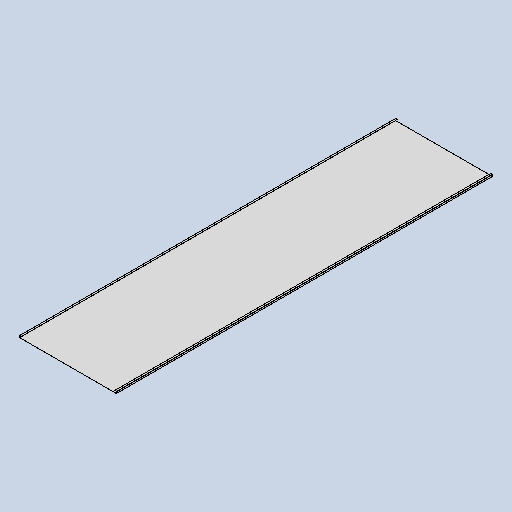
# Autodesk Inventor part: MSC 812 sheet gills
Saved by Autodesk Inventor 2025 (Build 290162010, 162A)
## iProperties
Created: 2024-06-15
Part Number: MSC 812 sheet gills
Material: Stainless Steel
Document SubType Name: Sheet Metal
Designer: pokla
Stock Number: МОО 0101 лист жабра
Mass: 8000 g
Surface Area: 40030 cm^2
Volume: 1000 cm^3
Density: 8 g/cm^3
Sheet Metal Rule: Default_mm
Appearance: Default
Author: pokla
Autodesk Inventor part; units mm, degrees
ref_plane "YZ Plane" through (0, 0, 0) normal (1, 0, 0) x (0, 1, 0)
ref_plane "XZ Plane" through (0, 0, 0) normal (0, 1, 0) x (-1, 0, 0)
ref_plane "XY Plane" through (0, 0, 0) normal (0, 0, 1) x (1, 0, 0)
sketch "Sketch6" plane through (0, 0, 0) normal (0, 1, 0) x (-1, 0, 0)
  line L0 (255.9, -990) -> (-255.9, -990)
  line L1 (-255.9, -990) -> (-255.9, 990)
  line L2 (-255.9, 990) -> (255.9, 990)
  line L3 (255.9, 990) -> (255.9, -990)
  line L4 (255.9, -990) -> (-255.9, 990) construction
  line L5 (-255.9, -990) -> (255.9, 990) construction
  point P0 (0, 0)
  dimension "d52" = 511.8
  dimension "d53" = 1980
  measures "d52" distance of L1.end L2.end
  measures "d53" distance of L0.end L1.end
extrude "Plate2" add sketch "Sketch6" along normal blind 0.5
sketch "Sketch12" plane through (255.4, 0, -990) normal (1, 0, 0) x (0, 1, 0)
  line L0 (0, 1980) -> (0, 0)
  line L1 (0, 0) -> (10, 0)
  line L2 (10, 0) -> (10, 1980)
  line L3 (10, 1980) -> (0, 1980)
  constraints: 6 end point, 1 horizontal, 1 perpendicular, 1 vertical
edge flange "Flange3" height 10 angle 90 thickness 0.5 bend radius 0.5 thickness toward (1, 0, 0) relief straight relief width 0.5 relief depth 0.25 edges at (255.9, 0.5, 0) wall of the first edge with corners at (255.4, 0, 990) (255.4, 0, -990) (255.4, 10, -990) (255.4, 10, 990)
bend "Bend4"
corner "Corner4"
sketch "Sketch13" plane through (255.9, 9.5, -990) normal (0, 1, 0) x (-1, 0, 0)
  line L0 (0, 1980) -> (0, 0)
  line L1 (0, 0) -> (10, 0)
  line L2 (10, 0) -> (10, 1980)
  line L3 (10, 1980) -> (0, 1980)
  constraints: 6 end point, 1 horizontal, 1 perpendicular, 1 vertical
edge flange "Flange4" height 10 angle 90 thickness 0.5 bend radius 0.5 thickness toward (0, 1, 0) relief straight relief width 0.5 relief depth 0.25 edges at (255.4, 10, 0) wall of the first edge with corners at (255.9, 9.5, 990) (255.9, 9.5, -990) (245.9, 9.5, -990) (245.9, 9.5, 990)
bend "Bend5"
corner "Corner5"
sketch "Sketch14" plane through (-255.4, 0, 990) normal (-1, 0, 0) x (0, -1, 0)
  line L0 (0, -1980) -> (0, 0)
  line L1 (0, 0) -> (-10, 0)
  line L2 (-10, 0) -> (-10, -1980)
  line L3 (-10, -1980) -> (0, -1980)
  constraints: 6 end point, 1 horizontal, 1 perpendicular, 1 vertical
edge flange "Flange5" height 10 angle 90 thickness 0.5 bend radius 0.5 thickness toward (-1, 0, 0) relief straight relief width 0.5 relief depth 0.25 edges at (-255.9, 0.5, 0) wall of the first edge with corners at (-255.4, 0, -990) (-255.4, 0, 990) (-255.4, 10, 990) (-255.4, 10, -990)
bend "Bend6"
corner "Corner6"
sketch "Sketch15" plane through (-255.9, 9.5, 990) normal (0, 1, 0) x (-1, 0, 0)
  line L0 (0, -1980) -> (0, 0)
  line L1 (0, 0) -> (-10, 0)
  line L2 (-10, 0) -> (-10, -1980)
  line L3 (-10, -1980) -> (0, -1980)
  constraints: 6 end point, 1 horizontal, 1 perpendicular, 1 vertical
edge flange "Flange6" height 10 angle 90 thickness 0.5 bend radius 0.5 thickness toward (0, 1, 0) relief straight relief width 0.5 relief depth 0.25 edges at (-255.4, 10, 0) wall of the first edge with corners at (-255.9, 9.5, -990) (-255.9, 9.5, 990) (-245.9, 9.5, 990) (-245.9, 9.5, -990)
bend "Bend7"
corner "Corner7"
equation "\"d52\" = ЖАБРЫ_базовая_ширина - 4 * ЖАБРЫ_шаг_листов"
equation "\"d53\" = ЖАБРЫ_базовая_длина_дл_лист"
equation "\"d54\" = Thickness"
equation "\"d94\" = BendReliefWidth"
equation "\"d95\" = BendReliefDepth"
equation "\"d96\" = MinimumRemnant"
equation "\"d97\" = TransitionRadius"
equation "\"d100\" = BendRadius"
equation "\"d101\" = CornerReliefSize"
equation "\"d102\" = GapSize"
equation "\"d103\" = JacobiRadiusSize"
equation "\"d104\" = BendReliefWidth"
equation "\"d105\" = BendReliefDepth"
equation "\"d106\" = MinimumRemnant"
equation "\"d107\" = TransitionRadius"
equation "\"d110\" = BendRadius"
equation "\"d111\" = CornerReliefSize"
equation "\"d112\" = GapSize"
equation "\"d113\" = JacobiRadiusSize"
equation "\"d114\" = BendReliefWidth"
equation "\"d115\" = BendReliefDepth"
equation "\"d116\" = MinimumRemnant"
equation "\"d117\" = TransitionRadius"
equation "\"d120\" = BendRadius"
equation "\"d121\" = CornerReliefSize"
equation "\"d122\" = GapSize"
equation "\"d123\" = JacobiRadiusSize"
equation "\"d124\" = BendReliefWidth"
equation "\"d125\" = BendReliefDepth"
equation "\"d126\" = MinimumRemnant"
equation "\"d127\" = TransitionRadius"
equation "\"d130\" = BendRadius"
equation "\"d131\" = CornerReliefSize"
equation "\"d132\" = GapSize"
equation "\"d133\" = JacobiRadiusSize"
equation "\"BendRadius\" = Thickness"
equation "\"BendReliefWidth\" = Thickness"
equation "\"BendReliefDepth\" = 0.5 * Thickness"
equation "\"CornerReliefSize\" = 4 * Thickness"
equation "\"MinimumRemnant\" = 2 * Thickness"
equation "\"TransitionRadius\" = BendRadius"
equation "\"JacobiRadiusSize\" = BendRadius"
equation "\"GapSize\" = Thickness"
equation "\"ЖАБРЫ_базовая_ширина\" = 915"
equation "\"ЖАБРЫ_шаг_листов\" = 100.8"
equation "\"ЖАБРЫ_базовая_длина_дл_лист\" = 1980"
equation "\"Thickness\" = 0.5"
body "Solid2"
